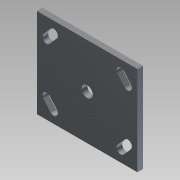
# Autodesk Inventor part: wheel mount plate
Saved by Autodesk Inventor 2013 (Build 170138000, 138)
## iProperties
Created: 2012-09-15
Part Number: wheel mount plate
Material: Generic
Document SubType Name: Modeling
Designer: Admin
Density: 1 g/cm^3
Author: Admin
Autodesk Inventor part; units mm, degrees
ref_plane "YZ Plane" through (0, 0, 0) normal (1, 0, 0) x (0, 1, 0)
ref_plane "XZ Plane" through (0, 0, 0) normal (0, 1, 0) x (-1, 0, 0)
ref_plane "XY Plane" through (0, 0, 0) normal (0, 0, 1) x (1, 0, 0)
sketch "Sketch1" plane through (0, 0, 0) normal (0, 0, 1) x (1, 0, 0)
  line L0 (0, 0) -> (-114.3, 0)
  line L1 (-114.3, 0) -> (-114.3, 101.6)
  line L2 (-114.3, 101.6) -> (0, 101.6)
  line L3 (0, 101.6) -> (0, 0)
  line L4 (0, 50.8) -> (0, 12.7)
  line L5 (0, 50.8) -> (0, 88.9)
  line L6 (-114.3, 50.8) -> (-114.3, 88.9)
  line L7 (-114.3, 50.8) -> (-114.3, 12.7)
  arc A0 (-92.4707, 85.033) -> (-98.8773, 91.9861) centre (-95.2491, 88.9011) ccw
  arc A1 (-15.4219, 91.9851) -> (-22.6777, 85.8144) centre (-19.05, 88.9) ccw
  arc A2 (-98.8781, 9.6149) -> (-91.6219, 15.7851) centre (-95.25, 12.7) ccw
  arc A3 (-22.6781, 15.7851) -> (-15.4219, 9.6149) centre (-19.05, 12.7) ccw
  line L8 (-57.15, 0) -> (-103.1875, 0)
  line L9 (-57.15, 0) -> (-11.1125, 0)
  line L10 (-57.15, 101.6) -> (-103.1875, 101.6)
  line L11 (-57.15, 101.6) -> (-11.1125, 101.6)
  arc A4 (-99.5594, 25.1196) -> (-106.8156, 18.9494) centre (-103.1875, 22.0345) ccw
  arc A5 (-7.4844, 18.9494) -> (-14.7406, 25.1196) centre (-11.1125, 22.0345) ccw
  arc A6 (-106.8154, 82.6503) -> (-99.5202, 76.5264) centre (-103.1872, 79.5653) ccw
  arc A7 (-14.7386, 76.4804) -> (-7.4832, 82.6517) centre (-11.1109, 79.5661) ccw
  line L12 (-90.9324, 86.8892) -> (-99.5202, 76.5264)
  line L13 (-106.8154, 82.6503) -> (-98.8773, 91.9861)
  line L14 (-15.4227, 91.9861) -> (-7.4832, 82.6517)
  line L15 (-14.7386, 76.4804) -> (-22.6777, 85.8144)
  line L16 (-14.7406, 25.1196) -> (-22.6781, 15.7851)
  line L17 (-15.4219, 9.6149) -> (-7.4844, 18.9494)
  line L18 (-99.5594, 25.1196) -> (-91.6219, 15.7851)
  line L19 (-106.8156, 18.9494) -> (-98.8781, 9.6149)
  dimension "d0" = 114.3
  dimension "d1" = 101.6
  dimension "d8" = 9.525
  dimension "d9" = 9.525
  dimension "d10" = 9.525
  dimension "d11" = 46.0375
  dimension "d14" = 46.0375
  dimension "d16" = 9.525
  dimension "d20" = 9.525
  dimension "d22" = 9.525
  constraints: 40 end point, 18 point on circle, 13 tangent, 10 point on line, 8 centre point, 4 midpoint, 2 perpendicular, 1 horizontal, 1 parallel
  measures "d0" distance of L0.start L0.end
  measures "d1" distance of L0.end L1.end
  measures "d8" diameter of A1
  measures "d9" diameter of A2
  measures "d10" diameter of A3
  measures "d11" distance of L8.start L8.end
  measures "d14" distance of L10.start L11.end
  measures "d16" diameter of A4
  measures "d20" diameter of A6
  measures "d22" diameter of A7
extrude "Extrusion1" add sketch "Sketch1" along normal blind 6.35
sketch "Sketch2" plane through (0, 0, 0) normal (0, 0, -1) x (-1, 0, 0)
  line L0 (0, 101.6) -> (114.3, 101.6) projected
  line L1 (0, 101.6) -> (57.15, 101.6)
  line L2 (57.15, 101.6) -> (57.15, 50.8)
  circle A0 centre (57.15, 50.8) radius 6.35
  dimension "d25" = 12.7
  constraints: 4 end point, 1 centre point, 1 coincident, 1 midpoint, 1 perpendicular
  measures "d25" diameter of A0
extrude "Extrusion2" cut sketch "Sketch2" against normal blind 6.35
body "Solid1"
